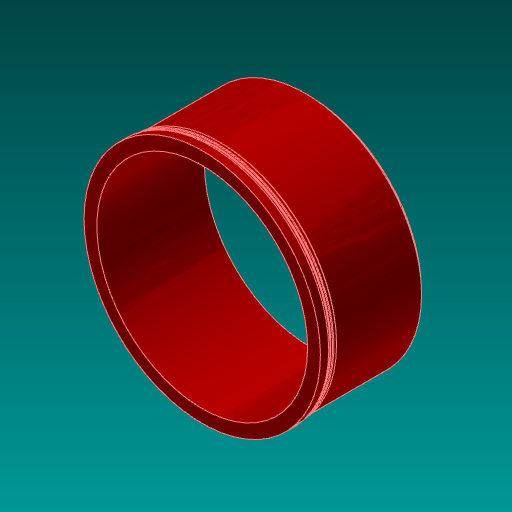
# Autodesk Inventor part: A1-19037-300-06 HCWI liner - pup
Saved by Autodesk Inventor 2017.3 (Build 213256000, 256)
## iProperties
Created: 2019-08-22
Part Number: A1-19037-300-06 HCWI liner - pup
Material: Iron, HCWI
Document SubType Name: Modeling
Designer: GVD
Density: 7.33517 g/cm^3
Appearance: Iron Gray(1)
Project: A1-19037--CNUL Albian CST laterals
Mass: 152708 g
Surface Area: 14597 cm^2
Volume: 20818.6 cm^3
Constructed By: Graeme_Van_Dongen
Project Name: CST laterals
Author: GVD
Autodesk Inventor part; units mm, degrees
ref_plane "YZ Plane" through (0, 0, 0) normal (1, 0, 0) x (0, 1, 0)
ref_plane "XZ Plane" through (0, 0, 0) normal (0, 1, 0) x (-1, 0, 0)
ref_plane "XY Plane" through (0, 0, 0) normal (0, 0, 1) x (1, 0, 0)
sketch "Sketch1" plane through (0, 0, 0) normal (0, 0, 1) x (1, 0, 0)
  circle A0 centre (0, 0) radius 311.15
  circle A1 centre (0, 0) radius 342.9
  dimension "d0" = 622.3
  dimension "d1" = 685.8
  constraints: 2 centre point, 2 coincident
  measures "d0" diameter of A0
  measures "d1" diameter of A1
extrude "Extrusion1" add sketch "Sketch1" along normal blind 304.8
sketch "Sketch2" plane through (0, 0, 304.8) normal (0, 0, 1) x (1, 0, 0)
  circle A0 centre (0, 0) radius 342.9 projected
  circle A1 centre (0, 0) radius 345.821
  circle A2 centre (0, 0) radius 348.996
  dimension "d4" = 691.642
  dimension "d5" = 697.992
  constraints: 2 centre point, 2 coincident
  measures "d4" diameter of A1
  measures "d5" diameter of A2
extrude "Extrusion2" add sketch "Sketch2" against normal blind 50.8 contours A1
extrude "Extrusion3" add sketch "Sketch2" against normal blind 25.4 contours A2
chamfer "Chamfer1" distance 2.921 angle 45 1 edges at (-342.9, 0, 254)
sketch "Sketch3" plane through (0, 0, 0) normal (0, 0, -1) x (-1, 0, 0)
  circle A0 centre (0, 0) radius 329.946
  circle A1 centre (0, 0) radius 311.15 projected
  dimension "d13" = 659.892
  constraints: 1 centre point, 1 coincident
  measures "d13" diameter of A0
extrude "Extrusion4" add sketch "Sketch3" along normal blind 12.7
fillet "Fillet1" radius 0.7937 2 edges at (329.946, 0, 0) (-345.821, 0, 279.4)
chamfer "Chamfer2" distance 0.7937 angle 45 1 edges at (329.946, 0, -12.7)
chamfer "Chamfer3" distance 0.7937 angle 45 1 edges at (-348.996, 0, 279.4)
sketch "Sketch4" plane through (0, 0, 0) normal (1, 0, 0) x (0, 1, 0)
  line L0 (345.821, 278.6062) -> (345.821, 254) construction
  line L1 (-348.996, 304.8) -> (348.996, 304.8) construction
  line L2 (345.821, 273.05) -> (344.0409, 271.2699)
  arc A0 (344.0409, 271.2699) -> (342.646, 267.9023) centre (347.4085, 267.9023) ccw
  line L3 (342.646, 267.9023) -> (342.646, 267.0852)
  arc A1 (342.646, 267.0852) -> (344.0409, 263.7176) centre (347.4085, 267.0852) ccw
  line L4 (344.0409, 263.7176) -> (345.821, 261.9375)
  line L5 (345.821, 261.9375) -> (345.821, 273.05)
  line L6 (0, -60.96) -> (0, 365.76) projected
  point P0 (0, 0)
  dimension "d23" = 11.1125
  dimension "d24" = 3.175
  dimension "d25" = 4.7625
  dimension "d26" = 31.75
  dimension "d27" = 45
  constraints: 8 end point, 4 point on circle, 4 tangent, 2 centre point, 2 point on line, 1 collinear, 1 equal radius, 1 perpendicular, 1 vertical
  measures "d23" distance of L2.start L4.end
  measures "d24" distance between parallel lines of L5 L3
  measures "d25" radius of A1
  measures "d26" distance from line of L1 L2.start
  measures "d27" angle of L5 L4
revolve "Revolution1" cut sketch "Sketch4" angle 360 about axis through (0, 0, -10) along (0, 0, 1)
equation "\"d10\" = -0.5 * d1 + 0.5 * d4"
body "Solid1"
